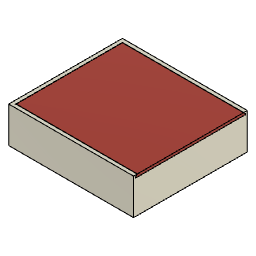
Battery Enclosure (Autodesk Fusion 360 archive; units mm, degrees)
design "Battery Enclosure" references "Battery Holder"
Autodesk Fusion 360 part; units mm, degrees
imported_body "Derived Base Feature" makes body 1
derive "ExternalDerived" from "Battery Holder v5"
sketch "Sketch8" plane through (0, 0, 0) normal (0, 0, 1) x (1, 0, 0)
  line L0 (63.5, 57.277) -> (0, 57.277)
  line L1 (63.5, 0) -> (63.5, 57.277)
  line L2 (0, 0) -> (63.5, 0)
  line L3 (-1, -1) -> (64.5, -1)
  line L4 (64.5, -1) -> (64.5, 58.277)
  line L5 (64.5, 58.277) -> (-1, 58.277)
  line L6 (-1, 58.277) -> (-1, -1)
  line L7 (0, 57.277) -> (0, 0)
  line L8 (66.5, -3) -> (-3, -3)
  line L9 (-3, -3) -> (-3, 60.277)
  line L10 (-3, 60.277) -> (66.5, 60.277)
  line L11 (66.5, 60.277) -> (66.5, -3)
  dimension "d27" = 1
  dimension "d28" = 1
  dimension "d29" = 1
  dimension "d30" = 1
  dimension "d31" = 2
  dimension "d32" = 2
  dimension "d33" = 2
  dimension "d34" = 2
  constraint horizontal L3
  constraint vertical L4
  constraint horizontal L5
  constraint vertical L6
  constraint horizontal L8
  constraint vertical L9
  constraint horizontal L10
  constraint vertical L11
  measures "d27" distance of L1 L4
  measures "d28" distance of L2 L3
  measures "d29" distance of L0 L5
  measures "d30" distance of L6 L7
  measures "d31" distance of L6 L9
  measures "d32" distance of L3 L8
  measures "d33" distance of L5 L10
  measures "d34" distance of L4 L11
extrude "Extrude3" add sketch "Sketch8" along normal blind 2 separate body contours L8 L9 L10 L11 makes body 2
extrude "Extrude4" add 1 faces at (42.6667, -2.3333, 2) along direction (0, 0, 1) blind 18 on bodies 2 bodies 2
sketch "Sketch11" plane through (0, -1, 0) normal (0, 1, 0) x (-1, 0, 0)
  line L0 (-64.5, 0) -> (1, 0)
  line L1 (1, 0) -> (1, 20)
  line L2 (1, 20) -> (-64.5, 20)
  line L3 (-64.5, 20) -> (-64.5, 0)
  line L4 (-64.5, 0) -> (1, 0)
  line L5 (1, 0) -> (1, 2)
  line L6 (1, 2) -> (-64.5, 2)
  line L7 (-64.5, 2) -> (-64.5, 0)
  dimension "d46" = 2
  constraint horizontal L4
  constraint vertical L5
  constraint horizontal L6
  constraint vertical L7
  constraint coincident L1 L5.end
  constraint coincident L0.start L3.end
  measures "d46" distance of L0.start L6.end
extrude "Extrude7" add sketch "Sketch11" along normal up to surface (59.277 mm away) contours L0 L1 L3 L4 L5 L6 L7 bodies 2
ref_plane "WorkPlane1" through (31.75, 28.6385, 18.5) normal (0, 0, 1) x (1, 0, 0)
sketch "Sketch12" plane through (31.75, 28.6385, 18.5) normal (0, 0, 1) x (1, 0, 0)
  line L0 (-33.75, 30.6385) -> (33.75, 30.6385)
  line L1 (33.75, 30.6385) -> (33.75, -30.6385)
  line L2 (33.75, -30.6385) -> (-33.75, -30.6385)
  line L3 (-33.75, -30.6385) -> (-33.75, 30.6385)
  line L4 (32.75, 29.6385) -> (32.75, -29.6385)
  line L5 (32.75, -29.6385) -> (-32.75, -29.6385)
  line L6 (-32.75, 29.6385) -> (32.75, 29.6385) construction
  line L7 (-32.75, -29.6385) -> (-32.75, 29.6385) construction
  line L8 (32.75, -29.6385) -> (-32.75, -29.6385) construction
  line L9 (-33.75, -30.6385) -> (-33.75, -41)
  line L10 (33.75, -30.6385) -> (33.75, -39.4017)
  dimension "d55" = 1
  dimension "d61" = 1
  constraint vertical L1
  constraint horizontal L2
  constraint vertical L3
  constraint vertical L4
  constraint horizontal L5
  constraint coincident L5 L4.end
  constraint coincident L4 L6.end
  constraint perpendicular L2 L9
  constraint perpendicular L2 L10
  measures "d55" distance of L1 L4
  measures "d61" distance of L0 L6
extrude "Extrude8" add sketch "Sketch12" along normal blind 1 separate body makes body 3
combine "Combine1" operation cut target body 2 tool bodies 3 keep tools
sketch "Sketch13" plane through (0, 0, 20) normal (0, 0, 1) x (-1, 0, 0)
  line L0 (1, 1) -> (1, -58.277)
  line L1 (1, -58.277) -> (-64.5, -58.277)
  line L2 (-64.5, -58.277) -> (-64.5, 1)
  line L3 (-64.5, 1) -> (1, 1)
  line L4 (-66.5, -60.277) -> (3, -60.277)
  line L5 (3, -60.277) -> (3, 3)
  line L6 (3, 3) -> (-66.5, 3)
  line L7 (-66.5, 3) -> (-66.5, -60.277)
  line L8 (-64.5, 1) -> (-69.7352, 1)
  line L9 (-64.5, -58.277) -> (-68, -58.277)
  constraint coincident L2.end L3.start
  constraint perpendicular L7 L8
  constraint coincident L1.end L2.start
  constraint perpendicular L2 L9
extrude "Extrude9" cut sketch "Sketch13" against normal blind 1.5 contours L2 L7 L8 L9 bodies 2
sketch "Sketch14" plane through (0, -1, 0) normal (0, 1, 0) x (-1, 0, 0)
  line L0 (-65.5, 19.5) -> (1, 19.5)
  line L1 (1, 19.5) -> (1, 20)
  line L2 (1, 20) -> (-66.5, 20)
  line L3 (-66.5, 20) -> (-66.5, 18.5)
  line L4 (-66.5, 18.5) -> (-65.5, 18.5)
  line L5 (-65.5, 18.5) -> (-65.5, 19.5)
  line L6 (-65.5, 19.5) -> (-66.5, 19.5)
  constraint coincident L0.start L5.end
  constraint coincident L3 L6.end
  constraint perpendicular L3 L6
extrude "Extrude10" cut sketch "Sketch14" against normal blind 1 contours L3 L4 L5 L6 bodies 2
extrude "Extrude11" cut 1 faces at (65.5, 58.9437, 18.8333) along direction (1, 0, 0) blind 1.8 on bodies 2 bodies 2
extrude "Extrude12" add 1 faces at (21.1667, -1.6667, 19.5) along direction (0, 0, -1) blind 0.5 on bodies 2 bodies 2
chamfer "Chamfer1" distance 1 angle 45 3 edges at (32.75, -1, 19) (-1, 28.6385, 19) (32.75, 58.277, 19) on bodies 2
extrude "Extrude13" add 1 faces at (65.5, 38.8513, 18.8333) along direction (1, 0, 0) up to surface (1 mm away) on bodies 3 bodies 3
extrude "Extrude14" add 1 faces at (43.6667, 18.4257, 19.5) along direction (0, 0, 1) blind 0.5 on bodies 3 bodies 3
chamfer "Chamfer2" distance 1.1 angle 45 3 edges at (32.25, -2, 20) (32.25, 59.277, 20) (-2, 28.6385, 20) on bodies 3
sketch "Sketch15" plane through (0, 0, 18.5) normal (0, 0, -1) x (1, 0, 0)
  line L0 (66.5, 2) -> (-2, 2)
  line L1 (-2, 2) -> (-2, -59.277)
  line L2 (-2, -59.277) -> (66.5, -59.277)
  line L3 (66.5, -59.277) -> (66.5, 2)
  line L4 (66.5, 1.9) -> (-1.9, 1.9)
  line L5 (-1.9, 1.9) -> (-1.9, -59.177)
  line L6 (-1.9, -59.177) -> (66.5, -59.177)
  line L7 (66.5, -59.177) -> (66.5, 1.9)
  dimension "d78" = 0.1
  dimension "d79" = 0.1
  dimension "d80" = 0.1
  constraint horizontal L4
  constraint vertical L5
  constraint horizontal L6
  constraint vertical L7
  constraint coincident L3 L4.start
  measures "d78" distance of L0 L4
  measures "d79" distance of L1 L5
  measures "d80" distance of L2 L6
extrude "Extrude15" cut sketch "Sketch15" against normal blind 60 contours L0 L1 L2 L3 L4 L5 L6 bodies 3
sketch "Sketch16" plane through (0, 60.277, 0) normal (0, 1, 0) x (-1, 0, 0)
  line L0 (-66.5, 0) -> (3, 0)
  line L1 (3, 0) -> (3, 20)
  line L2 (3, 20) -> (-66.5, 20)
  line L3 (-66.5, 20) -> (-66.5, 0)
  line L4 (-54.5, 6) -> (-47.5, 6)
  line L5 (-47.5, 6) -> (-47.5, 11)
  line L6 (-47.5, 11) -> (-54.5, 11)
  line L7 (-54.5, 11) -> (-54.5, 6)
  dimension "d83" = 7
  dimension "d84" = 5
  dimension "d85" = 12
  dimension "d86" = 9
  constraint horizontal L4
  constraint vertical L5
  constraint horizontal L6
  constraint vertical L7
  measures "d83" distance of L4.start L4.end
  measures "d84" distance of L4.start L6.end
  measures "d85" distance of L3 L7
  measures "d86" distance of L2 L6
extrude "Extrude16" cut sketch "Sketch16" against normal up to surface (2 mm away) contours L4 L5 L6 L7 bodies 2
hidden bodies 1
named bodies: "Body1"

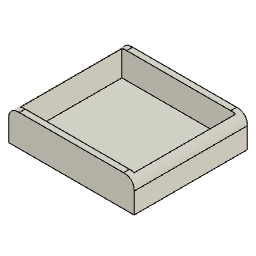
design "Battery Holder"
Autodesk Fusion 360 part; units mm, degrees
sketch "Sketch1" plane through (0, 0, 0) normal (0, 0, 1) x (1, 0, 0)
  line L0 (0, 0) -> (63.5, 0)
  line L1 (63.5, 0) -> (63.5, 57.277)
  line L2 (63.5, 57.277) -> (0, 57.277)
  line L3 (0, 57.277) -> (0, 0)
  dimension "d1" = 63.5
  dimension "d2" = 57.277
  constraint horizontal L0
  constraint vertical L1
  constraint horizontal L2
  constraint vertical L3
  constraint coincident L0.start L3.end
  measures "d1" distance of L0.start L0.end
  measures "d2" distance of L0.start L2.end
extrude "Extrude1" add sketch "Sketch1" along normal blind 15.875
sketch "Sketch2" plane through (0, 0, 15.875) normal (0, 0, 1) x (-1, 0, 0)
  line L0 (0, -57.277) -> (0, 0)
  line L1 (0, 0) -> (-63.5, 0)
  line L2 (-63.5, 0) -> (-63.5, -57.277)
  line L3 (-63.5, -57.277) -> (0, -57.277)
  line L4 (-60.5, -3) -> (-3, -3)
  line L5 (-3, -3) -> (-3, -54.277)
  line L6 (-3, -54.277) -> (-60.5, -54.277)
  line L7 (-60.5, -54.277) -> (-60.5, -3)
  dimension "d5" = 3
  dimension "d6" = 3
  dimension "d7" = 3
  dimension "d8" = 3
  dimension "d9" = 3
  constraint horizontal L4
  constraint perpendicular L4 L5
  constraint perpendicular L5 L6
  measures "d5" distance of L1 L4
  measures "d6" distance of L0 L4.end
  measures "d7" distance of L3 L5.end
  measures "d8" distance of L2 L4.start
  measures "d9" distance of L2 L6.end
extrude "Extrude2" cut sketch "Sketch2" against normal blind 13.156 contours L4 L5 L6 L7
fillet "Fillet1" chord length 7.62 curvature continuous 2 edges at (63.5, 28.6385, 15.875) (0, 28.6385, 15.875)
